Autodesk Fusion 360 part; units mm, degrees
note: some values were not read from the file. Chosen so that the rebuilt part matches the saved one: a direction. Set by a fixed rule: which sketch regions a step uses.
(part 4 of 5)
sketch "Sketch6" plane through (0, 0, 3.1479) normal (0, 0, 1) x (1, 0, 0)
  arc A0 (27.9575, -0.4591) -> (28.2196, 0.5192) centre (23.0613, 1.3771) ccw
  arc A1 (28.3326, 0.6018) -> (28.2196, 0.5192) centre (28.3182, 0.5028) ccw
  line L0 (28.3326, 0.6018) -> (29.1974, 0.4761)
  spline S0 degree 5 poles (29.1974, 0.4761) (29.2018, 0.4754) (29.2105, 0.4743) (29.2236, 0.473) (29.2412, 0.4721) (29.2633, 0.472) (29.2854, 0.4726) (29.3076, 0.4738) (29.3299, 0.4753) (29.3521, 0.4769) (29.3744, 0.4787) (29.3968, 0.4808) (29.4191, 0.4832) (29.4415, 0.486) (29.4639, 0.4891) (29.4863, 0.4927) (29.5087, 0.4965) (29.5311, 0.5006) (29.5536, 0.5049) (29.5761, 0.5095) (29.5985, 0.5143) (29.621, 0.5193) (29.6435, 0.5245) (29.666, 0.53) (29.6885, 0.5357) (29.711, 0.5417) (29.7335, 0.5479) (29.756, 0.5543) (29.7785, 0.561) (29.801, 0.5678) (29.8235, 0.5748) (29.846, 0.5821) (29.8684, 0.5895) (29.8909, 0.5972) (29.9134, 0.605) (29.9359, 0.6131) (29.9583, 0.6213) (29.9808, 0.6298) (30.0032, 0.6384) (30.0256, 0.6472) (30.048, 0.6562) (30.0704, 0.6654) (30.0928, 0.6748) (30.1152, 0.6843) (30.1375, 0.6941) (30.1598, 0.704) (30.1822, 0.7141) (30.2044, 0.7244) (30.2267, 0.7348) (30.249, 0.7455) (30.2712, 0.7563) (30.2934, 0.7672) (30.3156, 0.7784) (30.3378, 0.7897) (30.3599, 0.8012) (30.3821, 0.8128) (30.4042, 0.8246) (30.4262, 0.8366) (30.4483, 0.8488) (30.4703, 0.8611) (30.4923, 0.8736) (30.5142, 0.8862) (30.5362, 0.899) (30.5581, 0.912) (30.5799, 0.9251) (30.6018, 0.9384) (30.6236, 0.9518) (30.6454, 0.9654) (30.6671, 0.9791) (30.6888, 0.9931) (30.7105, 1.0071) (30.7278, 1.0185) (30.7407, 1.0271) (30.7494, 1.0329) (30.7537, 1.0357) knots 0 0 0 0 0 0 0.01428571 0.02857143 0.04285714 0.05714286 0.07142857 0.08571429 0.1 0.11428571 0.12857143 0.14285714 0.15714286 0.17142857 0.18571429 0.2 0.21428571 0.22857143 0.24285714 0.25714286 0.27142857 0.28571429 0.3 0.31428571 0.32857143 0.34285714 0.35714286 0.37142857 0.38571429 0.4 0.41428571 0.42857143 0.44285714 0.45714286 0.47142857 0.48571429 0.5 0.51428571 0.52857143 0.54285714 0.55714286 0.57142857 0.58571429 0.6 0.61428571 0.62857143 0.64285714 0.65714286 0.67142857 0.68571429 0.7 0.71428571 0.72857143 0.74285714 0.75714286 0.77142857 0.78571429 0.8 0.81428571 0.82857143 0.84285714 0.85714286 0.87142857 0.88571429 0.9 0.91428571 0.92857143 0.94285714 0.95714286 0.97142857 0.98571429 1 1 1 1 1 1
  arc A2 (30.7537, 1.0357) -> (30.7537, 1.7185) centre (23.0613, 1.3771) ccw
  spline S1 degree 5 poles (30.7537, 1.7185) (30.7494, 1.7214) (30.7407, 1.7272) (30.7278, 1.7358) (30.7105, 1.7471) (30.6888, 1.7612) (30.6671, 1.7751) (30.6454, 1.7889) (30.6236, 1.8025) (30.6018, 1.8159) (30.5799, 1.8292) (30.5581, 1.8423) (30.5362, 1.8553) (30.5142, 1.8681) (30.4923, 1.8807) (30.4703, 1.8932) (30.4483, 1.9055) (30.4262, 1.9176) (30.4042, 1.9296) (30.3821, 1.9414) (30.3599, 1.9531) (30.3378, 1.9646) (30.3156, 1.9759) (30.2934, 1.987) (30.2712, 1.998) (30.249, 2.0088) (30.2267, 2.0194) (30.2044, 2.0299) (30.1822, 2.0401) (30.1598, 2.0502) (30.1375, 2.0602) (30.1152, 2.0699) (30.0928, 2.0795) (30.0704, 2.0888) (30.048, 2.098) (30.0256, 2.107) (30.0032, 2.1159) (29.9808, 2.1245) (29.9583, 2.1329) (29.9359, 2.1412) (29.9134, 2.1492) (29.8909, 2.1571) (29.8684, 2.1647) (29.846, 2.1722) (29.8235, 2.1794) (29.801, 2.1864) (29.7785, 2.1933) (29.756, 2.1999) (29.7335, 2.2063) (29.711, 2.2125) (29.6885, 2.2185) (29.666, 2.2242) (29.6435, 2.2297) (29.621, 2.235) (29.5985, 2.24) (29.5761, 2.2448) (29.5536, 2.2493) (29.5311, 2.2536) (29.5087, 2.2577) (29.4863, 2.2616) (29.4639, 2.2651) (29.4415, 2.2683) (29.4191, 2.2711) (29.3968, 2.2735) (29.3744, 2.2755) (29.3521, 2.2774) (29.3299, 2.279) (29.3076, 2.2804) (29.2854, 2.2816) (29.2633, 2.2823) (29.2412, 2.2822) (29.2236, 2.2813) (29.2105, 2.28) (29.2018, 2.2788) (29.1974, 2.2782) knots -1 -1 -1 -1 -1 -1 -0.98571429 -0.97142857 -0.95714286 -0.94285714 -0.92857143 -0.91428571 -0.9 -0.88571429 -0.87142857 -0.85714286 -0.84285714 -0.82857143 -0.81428571 -0.8 -0.78571429 -0.77142857 -0.75714286 -0.74285714 -0.72857143 -0.71428571 -0.7 -0.68571429 -0.67142857 -0.65714286 -0.64285714 -0.62857143 -0.61428571 -0.6 -0.58571429 -0.57142857 -0.55714286 -0.54285714 -0.52857143 -0.51428571 -0.5 -0.48571429 -0.47142857 -0.45714286 -0.44285714 -0.42857143 -0.41428571 -0.4 -0.38571429 -0.37142857 -0.35714286 -0.34285714 -0.32857143 -0.31428571 -0.3 -0.28571429 -0.27142857 -0.25714286 -0.24285714 -0.22857143 -0.21428571 -0.2 -0.18571429 -0.17142857 -0.15714286 -0.14285714 -0.12857143 -0.11428571 -0.1 -0.08571429 -0.07142857 -0.05714286 -0.04285714 -0.02857143 -0.01428571 0 0 0 0 0 0
  line L1 (29.1974, 2.2782) -> (28.3326, 2.1525)
  arc A3 (28.2196, 2.2351) -> (28.3326, 2.1525) centre (28.3182, 2.2515) ccw
  arc A4 (28.2196, 2.2351) -> (27.9575, 3.2133) centre (23.0613, 1.3771) ccw
  arc A5 (28.0141, 3.3413) -> (27.9575, 3.2133) centre (28.0511, 3.2484) ccw
  line L2 (28.0141, 3.3413) -> (28.8259, 3.6649)
  spline S2 degree 5 poles (28.8259, 3.6649) (28.83, 3.6665) (28.8381, 3.6699) (28.8501, 3.6753) (28.8658, 3.6833) (28.885, 3.6943) (28.9038, 3.7059) (28.9224, 3.718) (28.941, 3.7304) (28.9594, 3.7429) (28.9778, 3.7557) (28.9961, 3.7686) (29.0143, 3.7819) (29.0323, 3.7955) (29.0501, 3.8094) (29.0677, 3.8237) (29.0852, 3.8382) (29.1026, 3.853) (29.1199, 3.868) (29.1371, 3.8831) (29.1541, 3.8985) (29.1711, 3.9141) (29.1879, 3.9299) (29.2047, 3.9459) (29.2213, 3.9621) (29.2378, 3.9785) (29.2542, 3.9951) (29.2704, 4.0119) (29.2866, 4.0289) (29.3027, 4.0461) (29.3186, 4.0634) (29.3345, 4.081) (29.3502, 4.0986) (29.3659, 4.1165) (29.3814, 4.1345) (29.3969, 4.1527) (29.4122, 4.1711) (29.4274, 4.1896) (29.4425, 4.2083) (29.4575, 4.2272) (29.4724, 4.2462) (29.4872, 4.2653) (29.5019, 4.2847) (29.5165, 4.3041) (29.531, 4.3237) (29.5454, 4.3435) (29.5596, 4.3634) (29.5738, 4.3834) (29.5879, 4.4036) (29.6018, 4.424) (29.6157, 4.4444) (29.6295, 4.465) (29.6431, 4.4858) (29.6566, 4.5067) (29.6701, 4.5277) (29.6834, 4.5488) (29.6966, 4.5701) (29.7098, 4.5915) (29.7228, 4.6131) (29.7357, 4.6347) (29.7485, 4.6565) (29.7612, 4.6785) (29.7738, 4.7005) (29.7863, 4.7227) (29.7986, 4.745) (29.8109, 4.7674) (29.8231, 4.7899) (29.8351, 4.8126) (29.8471, 4.8354) (29.8589, 4.8583) (29.8707, 4.8813) (29.88, 4.8998) (29.8869, 4.9137) (29.8915, 4.923) (29.8938, 4.9277) knots 0 0 0 0 0 0 0.01428571 0.02857143 0.04285714 0.05714286 0.07142857 0.08571429 0.1 0.11428571 0.12857143 0.14285714 0.15714286 0.17142857 0.18571429 0.2 0.21428571 0.22857143 0.24285714 0.25714286 0.27142857 0.28571429 0.3 0.31428571 0.32857143 0.34285714 0.35714286 0.37142857 0.38571429 0.4 0.41428571 0.42857143 0.44285714 0.45714286 0.47142857 0.48571429 0.5 0.51428571 0.52857143 0.54285714 0.55714286 0.57142857 0.58571429 0.6 0.61428571 0.62857143 0.64285714 0.65714286 0.67142857 0.68571429 0.7 0.71428571 0.72857143 0.74285714 0.75714286 0.77142857 0.78571429 0.8 0.81428571 0.82857143 0.84285714 0.85714286 0.87142857 0.88571429 0.9 0.91428571 0.92857143 0.94285714 0.95714286 0.97142857 0.98571429 1 1 1 1 1 1
  arc A6 (29.8938, 4.9277) -> (29.5524, 5.519) centre (23.0613, 1.3771) ccw
  spline S3 degree 5 poles (29.5524, 5.519) (29.5472, 5.5193) (29.5369, 5.52) (29.5213, 5.521) (29.5007, 5.5222) (29.4749, 5.5235) (29.4491, 5.5247) (29.4234, 5.5257) (29.3978, 5.5266) (29.3722, 5.5274) (29.3466, 5.528) (29.3211, 5.5284) (29.2957, 5.5287) (29.2703, 5.5288) (29.2449, 5.5287) (29.2197, 5.5286) (29.1944, 5.5282) (29.1693, 5.5277) (29.1442, 5.5271) (29.1191, 5.5262) (29.0941, 5.5253) (29.0692, 5.5241) (29.0444, 5.5228) (29.0196, 5.5214) (28.9948, 5.5198) (28.9702, 5.518) (28.9456, 5.5161) (28.9211, 5.514) (28.8966, 5.5118) (28.8722, 5.5094) (28.8479, 5.5068) (28.8237, 5.504) (28.7996, 5.5011) (28.7755, 5.4981) (28.7515, 5.4948) (28.7276, 5.4914) (28.7038, 5.4878) (28.68, 5.4841) (28.6564, 5.4802) (28.6328, 5.4761) (28.6093, 5.4718) (28.5859, 5.4674) (28.5627, 5.4628) (28.5395, 5.458) (28.5164, 5.453) (28.4934, 5.4479) (28.4705, 5.4426) (28.4477, 5.437) (28.425, 5.4314) (28.4024, 5.4255) (28.3799, 5.4194) (28.3576, 5.4131) (28.3353, 5.4066) (28.3132, 5.3999) (28.2913, 5.393) (28.2694, 5.3859) (28.2477, 5.3786) (28.2261, 5.3712) (28.2046, 5.3635) (28.1832, 5.3556) (28.1621, 5.3474) (28.1411, 5.339) (28.1203, 5.3302) (28.0998, 5.3211) (28.0794, 5.3118) (28.0592, 5.3022) (28.0391, 5.2925) (28.0191, 5.2826) (27.9993, 5.2725) (27.9798, 5.262) (27.9607, 5.2509) (27.946, 5.2413) (27.9352, 5.2336) (27.9282, 5.2283) (27.9248, 5.2256) knots -1 -1 -1 -1 -1 -1 -0.98571429 -0.97142857 -0.95714286 -0.94285714 -0.92857143 -0.91428571 -0.9 -0.88571429 -0.87142857 -0.85714286 -0.84285714 -0.82857143 -0.81428571 -0.8 -0.78571429 -0.77142857 -0.75714286 -0.74285714 -0.72857143 -0.71428571 -0.7 -0.68571429 -0.67142857 -0.65714286 -0.64285714 -0.62857143 -0.61428571 -0.6 -0.58571429 -0.57142857 -0.55714286 -0.54285714 -0.52857143 -0.51428571 -0.5 -0.48571429 -0.47142857 -0.45714286 -0.44285714 -0.42857143 -0.41428571 -0.4 -0.38571429 -0.37142857 -0.35714286 -0.34285714 -0.32857143 -0.31428571 -0.3 -0.28571429 -0.27142857 -0.25714286 -0.24285714 -0.22857143 -0.21428571 -0.2 -0.18571429 -0.17142857 -0.15714286 -0.14285714 -0.12857143 -0.11428571 -0.1 -0.08571429 -0.07142857 -0.05714286 -0.04285714 -0.02857143 -0.01428571 0 0 0 0 0 0
  line L3 (27.9248, 5.2256) -> (27.2387, 4.6843)
  arc A7 (27.0995, 4.6993) -> (27.2387, 4.6843) centre (27.1768, 4.7628) ccw
  arc A8 (27.0995, 4.6993) -> (26.3834, 5.4154) centre (23.0613, 1.3771) ccw
  arc A9 (26.3684, 5.5546) -> (26.3834, 5.4154) centre (26.4469, 5.4926) ccw
  line L4 (26.3684, 5.5546) -> (26.9097, 6.2407)
  spline S4 degree 5 poles (26.9097, 6.2407) (26.9124, 6.2441) (26.9178, 6.2511) (26.9254, 6.2619) (26.935, 6.2766) (26.9462, 6.2957) (26.9566, 6.3152) (26.9667, 6.335) (26.9766, 6.355) (26.9863, 6.3751) (26.9959, 6.3953) (27.0053, 6.4157) (27.0144, 6.4362) (27.0231, 6.457) (27.0316, 6.4779) (27.0397, 6.4991) (27.0476, 6.5205) (27.0553, 6.542) (27.0628, 6.5636) (27.07, 6.5853) (27.0771, 6.6071) (27.0841, 6.6291) (27.0908, 6.6512) (27.0972, 6.6734) (27.1035, 6.6958) (27.1096, 6.7183) (27.1155, 6.7408) (27.1212, 6.7635) (27.1267, 6.7863) (27.132, 6.8092) (27.1372, 6.8322) (27.1421, 6.8553) (27.1469, 6.8785) (27.1515, 6.9018) (27.156, 6.9252) (27.1602, 6.9487) (27.1643, 6.9723) (27.1682, 6.9959) (27.172, 7.0197) (27.1755, 7.0435) (27.179, 7.0674) (27.1822, 7.0914) (27.1853, 7.1154) (27.1882, 7.1396) (27.1909, 7.1638) (27.1935, 7.1881) (27.1959, 7.2125) (27.1981, 7.2369) (27.2002, 7.2615) (27.2022, 7.2861) (27.2039, 7.3107) (27.2055, 7.3354) (27.207, 7.3602) (27.2083, 7.3851) (27.2094, 7.41) (27.2104, 7.435) (27.2112, 7.46) (27.2118, 7.4851) (27.2123, 7.5103) (27.2127, 7.5355) (27.2129, 7.5608) (27.2129, 7.5861) (27.2128, 7.6115) (27.2125, 7.637) (27.2121, 7.6625) (27.2115, 7.688) (27.2108, 7.7136) (27.2099, 7.7393) (27.2088, 7.765) (27.2076, 7.7907) (27.2063, 7.8165) (27.2051, 7.8372) (27.2041, 7.8527) (27.2035, 7.8631) (27.2031, 7.8683) knots 0 0 0 0 0 0 0.01428571 0.02857143 0.04285714 0.05714286 0.07142857 0.08571429 0.1 0.11428571 0.12857143 0.14285714 0.15714286 0.17142857 0.18571429 0.2 0.21428571 0.22857143 0.24285714 0.25714286 0.27142857 0.28571429 0.3 0.31428571 0.32857143 0.34285714 0.35714286 0.37142857 0.38571429 0.4 0.41428571 0.42857143 0.44285714 0.45714286 0.47142857 0.48571429 0.5 0.51428571 0.52857143 0.54285714 0.55714286 0.57142857 0.58571429 0.6 0.61428571 0.62857143 0.64285714 0.65714286 0.67142857 0.68571429 0.7 0.71428571 0.72857143 0.74285714 0.75714286 0.77142857 0.78571429 0.8 0.81428571 0.82857143 0.84285714 0.85714286 0.87142857 0.88571429 0.9 0.91428571 0.92857143 0.94285714 0.95714286 0.97142857 0.98571429 1 1 1 1 1 1
  arc A10 (27.2031, 7.8683) -> (26.6118, 8.2097) centre (23.0613, 1.3771) ccw
  spline S5 degree 5 poles (26.6118, 8.2097) (26.6072, 8.2074) (26.5978, 8.2028) (26.5839, 8.1958) (26.5654, 8.1865) (26.5424, 8.1748) (26.5195, 8.163) (26.4967, 8.151) (26.4741, 8.139) (26.4515, 8.1268) (26.4291, 8.1145) (26.4068, 8.1021) (26.3846, 8.0897) (26.3626, 8.0771) (26.3407, 8.0644) (26.3189, 8.0516) (26.2972, 8.0387) (26.2757, 8.0256) (26.2542, 8.0125) (26.233, 7.9993) (26.2118, 7.986) (26.1908, 7.9725) (26.1699, 7.959) (26.1492, 7.9453) (26.1286, 7.9316) (26.1081, 7.9177) (26.0877, 7.9038) (26.0676, 7.8897) (26.0475, 7.8755) (26.0276, 7.8612) (26.0078, 7.8469) (25.9882, 7.8324) (25.9688, 7.8178) (25.9495, 7.8031) (25.9303, 7.7883) (25.9113, 7.7734) (25.8925, 7.7584) (25.8738, 7.7433) (25.8552, 7.728) (25.8369, 7.7127) (25.8187, 7.6973) (25.8006, 7.6818) (25.7828, 7.6661) (25.7651, 7.6504) (25.7476, 7.6345) (25.7302, 7.6186) (25.7131, 7.6025) (25.6961, 7.5863) (25.6793, 7.57) (25.6626, 7.5537) (25.6462, 7.5372) (25.63, 7.5206) (25.614, 7.5038) (25.5982, 7.487) (25.5826, 7.47) (25.5673, 7.4529) (25.5521, 7.4357) (25.5371, 7.4185) (25.5223, 7.4011) (25.5078, 7.3836) (25.4935, 7.3659) (25.4796, 7.3481) (25.466, 7.3302) (25.4527, 7.312) (25.4398, 7.2937) (25.4271, 7.2753) (25.4145, 7.2569) (25.4022, 7.2383) (25.39, 7.2197) (25.3784, 7.2008) (25.3674, 7.1817) (25.3595, 7.166) (25.354, 7.154) (25.3506, 7.1458) (25.349, 7.1417) knots -1 -1 -1 -1 -1 -1 -0.98571429 -0.97142857 -0.95714286 -0.94285714 -0.92857143 -0.91428571 -0.9 -0.88571429 -0.87142857 -0.85714286 -0.84285714 -0.82857143 -0.81428571 -0.8 -0.78571429 -0.77142857 -0.75714286 -0.74285714 -0.72857143 -0.71428571 -0.7 -0.68571429 -0.67142857 -0.65714286 -0.64285714 -0.62857143 -0.61428571 -0.6 -0.58571429 -0.57142857 -0.55714286 -0.54285714 -0.52857143 -0.51428571 -0.5 -0.48571429 -0.47142857 -0.45714286 -0.44285714 -0.42857143 -0.41428571 -0.4 -0.38571429 -0.37142857 -0.35714286 -0.34285714 -0.32857143 -0.31428571 -0.3 -0.28571429 -0.27142857 -0.25714286 -0.24285714 -0.22857143 -0.21428571 -0.2 -0.18571429 -0.17142857 -0.15714286 -0.14285714 -0.12857143 -0.11428571 -0.1 -0.08571429 -0.07142857 -0.05714286 -0.04285714 -0.02857143 -0.01428571 0 0 0 0 0 0
  line L5 (25.349, 7.1417) -> (25.0254, 6.33)
  arc A11 (24.8974, 6.2733) -> (25.0254, 6.33) centre (24.9326, 6.367) ccw
  arc A12 (24.8974, 6.2733) -> (23.9192, 6.5355) centre (23.0613, 1.3771) ccw
  arc A13 (23.8366, 6.6485) -> (23.9192, 6.5355) centre (23.9356, 6.6341) ccw
  line L6 (23.8366, 6.6485) -> (23.9623, 7.5133)
  spline S6 degree 5 poles (23.9623, 7.5133) (23.963, 7.5177) (23.9641, 7.5264) (23.9654, 7.5395) (23.9663, 7.5571) (23.9664, 7.5792) (23.9657, 7.6013) (23.9646, 7.6235) (23.9631, 7.6458) (23.9615, 7.668) (23.9597, 7.6903) (23.9576, 7.7126) (23.9552, 7.735) (23.9524, 7.7573) (23.9492, 7.7797) (23.9457, 7.8021) (23.9419, 7.8246) (23.9378, 7.847) (23.9334, 7.8695) (23.9289, 7.8919) (23.9241, 7.9144) (23.9191, 7.9369) (23.9139, 7.9594) (23.9084, 7.9819) (23.9026, 8.0044) (23.8967, 8.0269) (23.8905, 8.0494) (23.884, 8.0719) (23.8774, 8.0944) (23.8706, 8.1169) (23.8635, 8.1393) (23.8563, 8.1618) (23.8488, 8.1843) (23.8412, 8.2068) (23.8333, 8.2293) (23.8253, 8.2517) (23.817, 8.2742) (23.8086, 8.2966) (23.8, 8.3191) (23.7912, 8.3415) (23.7822, 8.3639) (23.773, 8.3863) (23.7636, 8.4087) (23.754, 8.431) (23.7443, 8.4534) (23.7344, 8.4757) (23.7243, 8.498) (23.714, 8.5203) (23.7035, 8.5426) (23.6929, 8.5649) (23.6821, 8.5871) (23.6711, 8.6093) (23.66, 8.6315) (23.6487, 8.6537) (23.6372, 8.6758) (23.6256, 8.6979) (23.6137, 8.72) (23.6018, 8.7421) (23.5896, 8.7642) (23.5773, 8.7862) (23.5648, 8.8082) (23.5522, 8.8301) (23.5394, 8.852) (23.5264, 8.8739) (23.5133, 8.8958) (23.5, 8.9177) (23.4866, 8.9395) (23.473, 8.9612) (23.4592, 8.983) (23.4453, 9.0047) (23.4313, 9.0263) (23.4199, 9.0436) (23.4113, 9.0566) (23.4055, 9.0652) (23.4026, 9.0696) knots 0 0 0 0 0 0 0.01428571 0.02857143 0.04285714 0.05714286 0.07142857 0.08571429 0.1 0.11428571 0.12857143 0.14285714 0.15714286 0.17142857 0.18571429 0.2 0.21428571 0.22857143 0.24285714 0.25714286 0.27142857 0.28571429 0.3 0.31428571 0.32857143 0.34285714 0.35714286 0.37142857 0.38571429 0.4 0.41428571 0.42857143 0.44285714 0.45714286 0.47142857 0.48571429 0.5 0.51428571 0.52857143 0.54285714 0.55714286 0.57142857 0.58571429 0.6 0.61428571 0.62857143 0.64285714 0.65714286 0.67142857 0.68571429 0.7 0.71428571 0.72857143 0.74285714 0.75714286 0.77142857 0.78571429 0.8 0.81428571 0.82857143 0.84285714 0.85714286 0.87142857 0.88571429 0.9 0.91428571 0.92857143 0.94285714 0.95714286 0.97142857 0.98571429 1 1 1 1 1 1
  arc A14 (23.4026, 9.0696) -> (22.7199, 9.0696) centre (23.0613, 1.3771) ccw
  spline S7 degree 5 poles (22.7199, 9.0696) (22.717, 9.0652) (22.7112, 9.0566) (22.7026, 9.0436) (22.6912, 9.0263) (22.6772, 9.0047) (22.6633, 8.983) (22.6495, 8.9612) (22.6359, 8.9395) (22.6225, 8.9177) (22.6092, 8.8958) (22.5961, 8.8739) (22.5831, 8.852) (22.5703, 8.8301) (22.5577, 8.8082) (22.5452, 8.7862) (22.5329, 8.7642) (22.5207, 8.7421) (22.5088, 8.72) (22.4969, 8.6979) (22.4853, 8.6758) (22.4738, 8.6537) (22.4625, 8.6315) (22.4514, 8.6093) (22.4404, 8.5871) (22.4296, 8.5649) (22.419, 8.5426) (22.4085, 8.5203) (22.3982, 8.498) (22.3881, 8.4757) (22.3782, 8.4534) (22.3685, 8.431) (22.3589, 8.4087) (22.3495, 8.3863) (22.3403, 8.3639) (22.3313, 8.3415) (22.3225, 8.3191) (22.3139, 8.2966) (22.3055, 8.2742) (22.2972, 8.2517) (22.2892, 8.2293) (22.2813, 8.2068) (22.2737, 8.1843) (22.2662, 8.1618) (22.259, 8.1393) (22.2519, 8.1169) (22.2451, 8.0944) (22.2385, 8.0719) (22.232, 8.0494) (22.2258, 8.0269) (22.2199, 8.0044) (22.2141, 7.9819) (22.2086, 7.9594) (22.2034, 7.9369) (22.1984, 7.9144) (22.1936, 7.8919) (22.1891, 7.8695) (22.1847, 7.847) (22.1806, 7.8246) (22.1768, 7.8021) (22.1733, 7.7797) (22.1701, 7.7573) (22.1673, 7.735) (22.1649, 7.7126) (22.1628, 7.6903) (22.161, 7.668) (22.1594, 7.6458) (22.1579, 7.6235) (22.1568, 7.6013) (22.1561, 7.5792) (22.1562, 7.5571) (22.1571, 7.5395) (22.1584, 7.5264) (22.1595, 7.5177) (22.1602, 7.5133) knots -1 -1 -1 -1 -1 -1 -0.98571429 -0.97142857 -0.95714286 -0.94285714 -0.92857143 -0.91428571 -0.9 -0.88571429 -0.87142857 -0.85714286 -0.84285714 -0.82857143 -0.81428571 -0.8 -0.78571429 -0.77142857 -0.75714286 -0.74285714 -0.72857143 -0.71428571 -0.7 -0.68571429 -0.67142857 -0.65714286 -0.64285714 -0.62857143 -0.61428571 -0.6 -0.58571429 -0.57142857 -0.55714286 -0.54285714 -0.52857143 -0.51428571 -0.5 -0.48571429 -0.47142857 -0.45714286 -0.44285714 -0.42857143 -0.41428571 -0.4 -0.38571429 -0.37142857 -0.35714286 -0.34285714 -0.32857143 -0.31428571 -0.3 -0.28571429 -0.27142857 -0.25714286 -0.24285714 -0.22857143 -0.21428571 -0.2 -0.18571429 -0.17142857 -0.15714286 -0.14285714 -0.12857143 -0.11428571 -0.1 -0.08571429 -0.07142857 -0.05714286 -0.04285714 -0.02857143 -0.01428571 0 0 0 0 0 0
  line L7 (22.1602, 7.5133) -> (22.2859, 6.6485)
  arc A15 (22.2033, 6.5355) -> (22.2859, 6.6485) centre (22.1869, 6.6341) ccw
  arc A16 (22.2033, 6.5355) -> (21.2251, 6.2733) centre (23.0613, 1.3771) ccw
  arc A17 (21.0971, 6.33) -> (21.2251, 6.2733) centre (21.19, 6.367) ccw
  line L8 (21.0971, 6.33) -> (20.7735, 7.1417)
  spline S8 degree 5 poles (20.7735, 7.1417) (20.7719, 7.1458) (20.7685, 7.154) (20.763, 7.166) (20.7551, 7.1817) (20.7441, 7.2008) (20.7325, 7.2197) (20.7203, 7.2383) (20.708, 7.2569) (20.6954, 7.2753) (20.6827, 7.2937) (20.6698, 7.312) (20.6565, 7.3302) (20.6429, 7.3481) (20.629, 7.3659) (20.6147, 7.3836) (20.6002, 7.4011) (20.5854, 7.4185) (20.5704, 7.4357) (20.5552, 7.4529) (20.5399, 7.47) (20.5243, 7.487) (20.5085, 7.5038) (20.4925, 7.5206) (20.4763, 7.5372) (20.4599, 7.5537) (20.4432, 7.57) (20.4264, 7.5863) (20.4094, 7.6025) (20.3923, 7.6186) (20.3749, 7.6345) (20.3574, 7.6504) (20.3397, 7.6661) (20.3219, 7.6818) (20.3038, 7.6973) (20.2856, 7.7127) (20.2673, 7.728) (20.2487, 7.7433) (20.23, 7.7584) (20.2112, 7.7734) (20.1922, 7.7883) (20.173, 7.8031) (20.1537, 7.8178) (20.1343, 7.8324) (20.1147, 7.8469) (20.0949, 7.8612) (20.075, 7.8755) (20.0549, 7.8897) (20.0348, 7.9038) (20.0144, 7.9177) (19.994, 7.9316) (19.9733, 7.9453) (19.9526, 7.959) (19.9317, 7.9725) (19.9107, 7.986) (19.8895, 7.9993) (19.8683, 8.0125) (19.8468, 8.0256) (19.8253, 8.0387) (19.8036, 8.0516) (19.7818, 8.0644) (19.7599, 8.0771) (19.7379, 8.0897) (19.7157, 8.1021) (19.6934, 8.1145) (19.671, 8.1268) (19.6484, 8.139) (19.6258, 8.151) (19.603, 8.163) (19.5801, 8.1748) (19.5571, 8.1865) (19.5386, 8.1958) (19.5247, 8.2028) (19.5153, 8.2074) (19.5107, 8.2097) knots 0 0 0 0 0 0 0.01428571 0.02857143 0.04285714 0.05714286 0.07142857 0.08571429 0.1 0.11428571 0.12857143 0.14285714 0.15714286 0.17142857 0.18571429 0.2 0.21428571 0.22857143 0.24285714 0.25714286 0.27142857 0.28571429 0.3 0.31428571 0.32857143 0.34285714 0.35714286 0.37142857 0.38571429 0.4 0.41428571 0.42857143 0.44285714 0.45714286 0.47142857 0.48571429 0.5 0.51428571 0.52857143 0.54285714 0.55714286 0.57142857 0.58571429 0.6 0.61428571 0.62857143 0.64285714 0.65714286 0.67142857 0.68571429 0.7 0.71428571 0.72857143 0.74285714 0.75714286 0.77142857 0.78571429 0.8 0.81428571 0.82857143 0.84285714 0.85714286 0.87142857 0.88571429 0.9 0.91428571 0.92857143 0.94285714 0.95714286 0.97142857 0.98571429 1 1 1 1 1 1
  arc A18 (19.5107, 8.2097) -> (18.9194, 7.8683) centre (23.0613, 1.3771) ccw
  spline S9 degree 5 poles (18.9194, 7.8683) (18.919, 7.8631) (18.9184, 7.8527) (18.9174, 7.8372) (18.9162, 7.8165) (18.9149, 7.7907) (18.9137, 7.765) (18.9126, 7.7393) (18.9117, 7.7136) (18.911, 7.688) (18.9104, 7.6625) (18.91, 7.637) (18.9097, 7.6115) (18.9096, 7.5861) (18.9096, 7.5608) (18.9098, 7.5355) (18.9102, 7.5103) (18.9107, 7.4851) (18.9113, 7.46) (18.9121, 7.435) (18.9131, 7.41) (18.9142, 7.3851) (18.9155, 7.3602) (18.917, 7.3354) (18.9186, 7.3107) (18.9203, 7.2861) (18.9223, 7.2615) (18.9244, 7.2369) (18.9266, 7.2125) (18.929, 7.1881) (18.9316, 7.1638) (18.9343, 7.1396) (18.9372, 7.1154) (18.9403, 7.0914) (18.9436, 7.0674) (18.947, 7.0435) (18.9505, 7.0197) (18.9543, 6.9959) (18.9582, 6.9723) (18.9623, 6.9487) (18.9665, 6.9252) (18.971, 6.9018) (18.9756, 6.8785) (18.9804, 6.8553) (18.9853, 6.8322) (18.9905, 6.8092) (18.9958, 6.7863) (19.0013, 6.7635) (19.007, 6.7408) (19.0129, 6.7183) (19.019, 6.6958) (19.0253, 6.6734) (19.0317, 6.6512) (19.0385, 6.6291) (19.0454, 6.6071) (19.0525, 6.5853) (19.0597, 6.5636) (19.0672, 6.542) (19.0749, 6.5205) (19.0828, 6.4991) (19.0909, 6.4779) (19.0994, 6.457) (19.1081, 6.4362) (19.1172, 6.4157) (19.1266, 6.3953) (19.1362, 6.3751) (19.1459, 6.355) (19.1558, 6.335) (19.1659, 6.3152) (19.1763, 6.2957) (19.1875, 6.2766) (19.1971, 6.2619) (19.2047, 6.2511) (19.2101, 6.2441) (19.2128, 6.2407) knots -1 -1 -1 -1 -1 -1 -0.98571429 -0.97142857 -0.95714286 -0.94285714 -0.92857143 -0.91428571 -0.9 -0.88571429 -0.87142857 -0.85714286 -0.84285714 -0.82857143 -0.81428571 -0.8 -0.78571429 -0.77142857 -0.75714286 -0.74285714 -0.72857143 -0.71428571 -0.7 -0.68571429 -0.67142857 -0.65714286 -0.64285714 -0.62857143 -0.61428571 -0.6 -0.58571429 -0.57142857 -0.55714286 -0.54285714 -0.52857143 -0.51428571 -0.5 -0.48571429 -0.47142857 -0.45714286 -0.44285714 -0.42857143 -0.41428571 -0.4 -0.38571429 -0.37142857 -0.35714286 -0.34285714 -0.32857143 -0.31428571 -0.3 -0.28571429 -0.27142857 -0.25714286 -0.24285714 -0.22857143 -0.21428571 -0.2 -0.18571429 -0.17142857 -0.15714286 -0.14285714 -0.12857143 -0.11428571 -0.1 -0.08571429 -0.07142857 -0.05714286 -0.04285714 -0.02857143 -0.01428571 0 0 0 0 0 0
  line L9 (19.2128, 6.2407) -> (19.7541, 5.5546)
  arc A19 (19.7391, 5.4154) -> (19.7541, 5.5546) centre (19.6756, 5.4926) ccw
  arc A20 (19.7391, 5.4154) -> (19.023, 4.6993) centre (23.0613, 1.3771) ccw
  arc A21 (18.8838, 4.6843) -> (19.023, 4.6993) centre (18.9457, 4.7628) ccw
  line L10 (18.8838, 4.6843) -> (18.1977, 5.2256)
  spline S10 degree 5 poles (18.1977, 5.2256) (18.1943, 5.2283) (18.1873, 5.2336) (18.1765, 5.2413) (18.1618, 5.2509) (18.1427, 5.262) (18.1232, 5.2725) (18.1034, 5.2826) (18.0834, 5.2925) (18.0633, 5.3022) (18.0431, 5.3118) (18.0227, 5.3211) (18.0022, 5.3302) (17.9814, 5.339) (17.9604, 5.3474) (17.9393, 5.3556) (17.9179, 5.3635) (17.8964, 5.3712) (17.8748, 5.3786) (17.8531, 5.3859) (17.8312, 5.393) (17.8093, 5.3999) (17.7872, 5.4066) (17.7649, 5.4131) (17.7426, 5.4194) (17.7201, 5.4255) (17.6975, 5.4314) (17.6748, 5.437) (17.652, 5.4426) (17.6291, 5.4479) (17.6061, 5.453) (17.583, 5.458) (17.5599, 5.4628) (17.5366, 5.4674) (17.5132, 5.4718) (17.4897, 5.4761) (17.4661, 5.4802) (17.4425, 5.4841) (17.4187, 5.4878) (17.3949, 5.4914) (17.371, 5.4948) (17.347, 5.4981) (17.3229, 5.5011) (17.2988, 5.504) (17.2746, 5.5068) (17.2503, 5.5094) (17.2259, 5.5118) (17.2014, 5.514) (17.1769, 5.5161) (17.1523, 5.518) (17.1277, 5.5198) (17.1029, 5.5214) (17.0782, 5.5228) (17.0533, 5.5241) (17.0284, 5.5253) (17.0034, 5.5262) (16.9783, 5.5271) (16.9532, 5.5277) (16.9281, 5.5282) (16.9029, 5.5286) (16.8776, 5.5287) (16.8522, 5.5288) (16.8268, 5.5287) (16.8014, 5.5284) (16.7759, 5.528) (16.7503, 5.5274) (16.7247, 5.5266) (16.6991, 5.5257) (16.6734, 5.5247) (16.6476, 5.5235) (16.6219, 5.5222) (16.6012, 5.521) (16.5856, 5.52) (16.5753, 5.5193) (16.5701, 5.519) knots 0 0 0 0 0 0 0.01428571 0.02857143 0.04285714 0.05714286 0.07142857 0.08571429 0.1 0.11428571 0.12857143 0.14285714 0.15714286 0.17142857 0.18571429 0.2 0.21428571 0.22857143 0.24285714 0.25714286 0.27142857 0.28571429 0.3 0.31428571 0.32857143 0.34285714 0.35714286 0.37142857 0.38571429 0.4 0.41428571 0.42857143 0.44285714 0.45714286 0.47142857 0.48571429 0.5 0.51428571 0.52857143 0.54285714 0.55714286 0.57142857 0.58571429 0.6 0.61428571 0.62857143 0.64285714 0.65714286 0.67142857 0.68571429 0.7 0.71428571 0.72857143 0.74285714 0.75714286 0.77142857 0.78571429 0.8 0.81428571 0.82857143 0.84285714 0.85714286 0.87142857 0.88571429 0.9 0.91428571 0.92857143 0.94285714 0.95714286 0.97142857 0.98571429 1 1 1 1 1 1
  arc A22 (16.5701, 5.519) -> (16.2287, 4.9277) centre (23.0613, 1.3771) ccw
  spline S11 degree 5 poles (16.2287, 4.9277) (16.231, 4.923) (16.2356, 4.9137) (16.2425, 4.8998) (16.2518, 4.8813) (16.2636, 4.8583) (16.2754, 4.8354) (16.2874, 4.8126) (16.2994, 4.7899) (16.3116, 4.7674) (16.3239, 4.745) (16.3362, 4.7227) (16.3487, 4.7005) (16.3613, 4.6785) (16.374, 4.6565) (16.3868, 4.6347) (16.3997, 4.6131) (16.4127, 4.5915) (16.4259, 4.5701) (16.4391, 4.5488) (16.4524, 4.5277) (16.4659, 4.5067) (16.4794, 4.4858) (16.493, 4.465) (16.5068, 4.4444) (16.5207, 4.424) (16.5346, 4.4036) (16.5487, 4.3834) (16.5629, 4.3634) (16.5771, 4.3435) (16.5915, 4.3237) (16.606, 4.3041) (16.6206, 4.2847) (16.6353, 4.2653) (16.6501, 4.2462) (16.665, 4.2272) (16.68, 4.2083) (16.6951, 4.1896) (16.7103, 4.1711) (16.7257, 4.1527) (16.7411, 4.1345) (16.7566, 4.1165) (16.7723, 4.0986) (16.788, 4.081) (16.8039, 4.0634) (16.8198, 4.0461) (16.8359, 4.0289) (16.8521, 4.0119) (16.8683, 3.9951) (16.8847, 3.9785) (16.9012, 3.9621) (16.9178, 3.9459) (16.9346, 3.9299) (16.9514, 3.9141) (16.9684, 3.8985) (16.9855, 3.8831) (17.0026, 3.868) (17.0199, 3.853) (17.0373, 3.8382) (17.0548, 3.8237) (17.0724, 3.8094) (17.0902, 3.7955) (17.1082, 3.7819) (17.1264, 3.7686) (17.1447, 3.7557) (17.1631, 3.7429) (17.1815, 3.7304) (17.2001, 3.718) (17.2187, 3.7059) (17.2375, 3.6943) (17.2567, 3.6833) (17.2724, 3.6753) (17.2844, 3.6699) (17.2925, 3.6665) (17.2966, 3.6649) knots -1 -1 -1 -1 -1 -1 -0.98571429 -0.97142857 -0.95714286 -0.94285714 -0.92857143 -0.91428571 -0.9 -0.88571429 -0.87142857 -0.85714286 -0.84285714 -0.82857143 -0.81428571 -0.8 -0.78571429 -0.77142857 -0.75714286 -0.74285714 -0.72857143 -0.71428571 -0.7 -0.68571429 -0.67142857 -0.65714286 -0.64285714 -0.62857143 -0.61428571 -0.6 -0.58571429 -0.57142857 -0.55714286 -0.54285714 -0.52857143 -0.51428571 -0.5 -0.48571429 -0.47142857 -0.45714286 -0.44285714 -0.42857143 -0.41428571 -0.4 -0.38571429 -0.37142857 -0.35714286 -0.34285714 -0.32857143 -0.31428571 -0.3 -0.28571429 -0.27142857 -0.25714286 -0.24285714 -0.22857143 -0.21428571 -0.2 -0.18571429 -0.17142857 -0.15714286 -0.14285714 -0.12857143 -0.11428571 -0.1 -0.08571429 -0.07142857 -0.05714286 -0.04285714 -0.02857143 -0.01428571 0 0 0 0 0 0
  line L11 (17.2966, 3.6649) -> (18.1084, 3.3413)
  arc A23 (18.165, 3.2133) -> (18.1084, 3.3413) centre (18.0714, 3.2484) ccw
  arc A24 (18.165, 3.2133) -> (17.9029, 2.2351) centre (23.0613, 1.3771) ccw
  arc A25 (17.7899, 2.1525) -> (17.9029, 2.2351) centre (17.8043, 2.2515) ccw
  line L12 (17.7899, 2.1525) -> (16.9251, 2.2782)
  spline S12 degree 5 poles (16.9251, 2.2782) (16.9207, 2.2788) (16.912, 2.28) (16.8989, 2.2813) (16.8813, 2.2822) (16.8592, 2.2823) (16.8371, 2.2816) (16.8149, 2.2804) (16.7926, 2.279) (16.7704, 2.2774) (16.7481, 2.2755) (16.7258, 2.2735) (16.7034, 2.2711) (16.681, 2.2683) (16.6587, 2.2651) (16.6362, 2.2616) (16.6138, 2.2577) (16.5914, 2.2536) (16.5689, 2.2493) (16.5464, 2.2448) (16.524, 2.24) (16.5015, 2.235) (16.479, 2.2297) (16.4565, 2.2242) (16.434, 2.2185) (16.4115, 2.2125) (16.389, 2.2063) (16.3665, 2.1999) (16.344, 2.1933) (16.3215, 2.1864) (16.299, 2.1794) (16.2765, 2.1722) (16.2541, 2.1647) (16.2316, 2.1571) (16.2091, 2.1492) (16.1867, 2.1412) (16.1642, 2.1329) (16.1418, 2.1245) (16.1193, 2.1159) (16.0969, 2.107) (16.0745, 2.098) (16.0521, 2.0888) (16.0297, 2.0795) (16.0073, 2.0699) (15.985, 2.0602) (15.9627, 2.0502) (15.9404, 2.0401) (15.9181, 2.0299) (15.8958, 2.0194) (15.8735, 2.0088) (15.8513, 1.998) (15.8291, 1.987) (15.8069, 1.9759) (15.7847, 1.9646) (15.7626, 1.9531) (15.7404, 1.9414) (15.7183, 1.9296) (15.6963, 1.9176) (15.6742, 1.9055) (15.6522, 1.8932) (15.6302, 1.8807) (15.6083, 1.8681) (15.5863, 1.8553) (15.5644, 1.8423) (15.5426, 1.8292) (15.5207, 1.8159) (15.4989, 1.8025) (15.4772, 1.7889) (15.4554, 1.7751) (15.4337, 1.7612) (15.412, 1.7471) (15.3947, 1.7358) (15.3818, 1.7272) (15.3731, 1.7214) (15.3688, 1.7185) knots 0 0 0 0 0 0 0.01428571 0.02857143 0.04285714 0.05714286 0.07142857 0.08571429 0.1 0.11428571 0.12857143 0.14285714 0.15714286 0.17142857 0.18571429 0.2 0.21428571 0.22857143 0.24285714 0.25714286 0.27142857 0.28571429 0.3 0.31428571 0.32857143 0.34285714 0.35714286 0.37142857 0.38571429 0.4 0.41428571 0.42857143 0.44285714 0.45714286 0.47142857 0.48571429 0.5 0.51428571 0.52857143 0.54285714 0.55714286 0.57142857 0.58571429 0.6 0.61428571 0.62857143 0.64285714 0.65714286 0.67142857 0.68571429 0.7 0.71428571 0.72857143 0.74285714 0.75714286 0.77142857 0.78571429 0.8 0.81428571 0.82857143 0.84285714 0.85714286 0.87142857 0.88571429 0.9 0.91428571 0.92857143 0.94285714 0.95714286 0.97142857 0.98571429 1 1 1 1 1 1
  arc A26 (15.3688, 1.7185) -> (15.3688, 1.0357) centre (23.0613, 1.3771) ccw
  spline S13 degree 5 poles (15.3688, 1.0357) (15.3731, 1.0329) (15.3818, 1.0271) (15.3947, 1.0185) (15.412, 1.0071) (15.4337, 0.9931) (15.4554, 0.9791) (15.4772, 0.9654) (15.4989, 0.9518) (15.5207, 0.9384) (15.5426, 0.9251) (15.5644, 0.912) (15.5863, 0.899) (15.6083, 0.8862) (15.6302, 0.8736) (15.6522, 0.8611) (15.6742, 0.8488) (15.6963, 0.8366) (15.7183, 0.8246) (15.7404, 0.8128) (15.7626, 0.8012) (15.7847, 0.7897) (15.8069, 0.7784) (15.8291, 0.7672) (15.8513, 0.7563) (15.8735, 0.7455) (15.8958, 0.7348) (15.9181, 0.7244) (15.9404, 0.7141) (15.9627, 0.704) (15.985, 0.6941) (16.0073, 0.6843) (16.0297, 0.6748) (16.0521, 0.6654) (16.0745, 0.6562) (16.0969, 0.6472) (16.1193, 0.6384) (16.1418, 0.6298) (16.1642, 0.6213) (16.1867, 0.6131) (16.2091, 0.605) (16.2316, 0.5972) (16.2541, 0.5895) (16.2765, 0.5821) (16.299, 0.5748) (16.3215, 0.5678) (16.344, 0.561) (16.3665, 0.5543) (16.389, 0.5479) (16.4115, 0.5417) (16.434, 0.5357) (16.4565, 0.53) (16.479, 0.5245) (16.5015, 0.5193) (16.524, 0.5143) (16.5464, 0.5095) (16.5689, 0.5049) (16.5914, 0.5006) (16.6138, 0.4965) (16.6362, 0.4927) (16.6587, 0.4891) (16.681, 0.486) (16.7034, 0.4832) (16.7258, 0.4808) (16.7481, 0.4787) (16.7704, 0.4769) (16.7926, 0.4753) (16.8149, 0.4738) (16.8371, 0.4726) (16.8592, 0.472) (16.8813, 0.4721) (16.8989, 0.473) (16.912, 0.4743) (16.9207, 0.4754) (16.9251, 0.4761) knots -1 -1 -1 -1 -1 -1 -0.98571429 -0.97142857 -0.95714286 -0.94285714 -0.92857143 -0.91428571 -0.9 -0.88571429 -0.87142857 -0.85714286 -0.84285714 -0.82857143 -0.81428571 -0.8 -0.78571429 -0.77142857 -0.75714286 -0.74285714 -0.72857143 -0.71428571 -0.7 -0.68571429 -0.67142857 -0.65714286 -0.64285714 -0.62857143 -0.61428571 -0.6 -0.58571429 -0.57142857 -0.55714286 -0.54285714 -0.52857143 -0.51428571 -0.5 -0.48571429 -0.47142857 -0.45714286 -0.44285714 -0.42857143 -0.41428571 -0.4 -0.38571429 -0.37142857 -0.35714286 -0.34285714 -0.32857143 -0.31428571 -0.3 -0.28571429 -0.27142857 -0.25714286 -0.24285714 -0.22857143 -0.21428571 -0.2 -0.18571429 -0.17142857 -0.15714286 -0.14285714 -0.12857143 -0.11428571 -0.1 -0.08571429 -0.07142857 -0.05714286 -0.04285714 -0.02857143 -0.01428571 0 0 0 0 0 0
  line L13 (16.9251, 0.4761) -> (17.7899, 0.6018)
  arc A27 (17.9029, 0.5192) -> (17.7899, 0.6018) centre (17.8043, 0.5028) ccw
  arc A28 (17.9029, 0.5192) -> (18.165, -0.4591) centre (23.0613, 1.3771) ccw
  arc A29 (18.1084, -0.5871) -> (18.165, -0.4591) centre (18.0714, -0.4942) ccw
  line L14 (18.1084, -0.5871) -> (17.2966, -0.9106)
  spline S14 degree 5 poles (17.2966, -0.9106) (17.2925, -0.9122) (17.2844, -0.9156) (17.2724, -0.9211) (17.2567, -0.9291) (17.2375, -0.94) (17.2187, -0.9517) (17.2001, -0.9638) (17.1815, -0.9761) (17.1631, -0.9887) (17.1447, -1.0014) (17.1264, -1.0144) (17.1082, -1.0276) (17.0902, -1.0412) (17.0724, -1.0551) (17.0548, -1.0694) (17.0373, -1.084) (17.0199, -1.0987) (17.0026, -1.1137) (16.9855, -1.1289) (16.9684, -1.1443) (16.9514, -1.1598) (16.9346, -1.1756) (16.9178, -1.1916) (16.9012, -1.2078) (16.8847, -1.2243) (16.8683, -1.2409) (16.8521, -1.2577) (16.8359, -1.2747) (16.8198, -1.2918) (16.8039, -1.3092) (16.788, -1.3267) (16.7723, -1.3444) (16.7566, -1.3623) (16.7411, -1.3803) (16.7257, -1.3985) (16.7103, -1.4169) (16.6951, -1.4354) (16.68, -1.4541) (16.665, -1.4729) (16.6501, -1.4919) (16.6353, -1.5111) (16.6206, -1.5304) (16.606, -1.5499) (16.5915, -1.5695) (16.5771, -1.5892) (16.5629, -1.6091) (16.5487, -1.6292) (16.5346, -1.6494) (16.5207, -1.6697) (16.5068, -1.6902) (16.493, -1.7108) (16.4794, -1.7315) (16.4659, -1.7524) (16.4524, -1.7734) (16.4391, -1.7946) (16.4259, -1.8159) (16.4127, -1.8373) (16.3997, -1.8588) (16.3868, -1.8805) (16.374, -1.9023) (16.3613, -1.9242) (16.3487, -1.9463) (16.3362, -1.9684) (16.3239, -1.9907) (16.3116, -2.0132) (16.2994, -2.0357) (16.2874, -2.0584) (16.2754, -2.0811) (16.2636, -2.104) (16.2518, -2.127) (16.2425, -2.1455) (16.2356, -2.1595) (16.231, -2.1688) (16.2287, -2.1734) knots 0 0 0 0 0 0 0.01428571 0.02857143 0.04285714 0.05714286 0.07142857 0.08571429 0.1 0.11428571 0.12857143 0.14285714 0.15714286 0.17142857 0.18571429 0.2 0.21428571 0.22857143 0.24285714 0.25714286 0.27142857 0.28571429 0.3 0.31428571 0.32857143 0.34285714 0.35714286 0.37142857 0.38571429 0.4 0.41428571 0.42857143 0.44285714 0.45714286 0.47142857 0.48571429 0.5 0.51428571 0.52857143 0.54285714 0.55714286 0.57142857 0.58571429 0.6 0.61428571 0.62857143 0.64285714 0.65714286 0.67142857 0.68571429 0.7 0.71428571 0.72857143 0.74285714 0.75714286 0.77142857 0.78571429 0.8 0.81428571 0.82857143 0.84285714 0.85714286 0.87142857 0.88571429 0.9 0.91428571 0.92857143 0.94285714 0.95714286 0.97142857 0.98571429 1 1 1 1 1 1
  arc A30 (16.2287, -2.1734) -> (16.5701, -2.7647) centre (23.0613, 1.3771) ccw
  spline S15 degree 5 poles (16.5701, -2.7647) (16.5753, -2.7651) (16.5856, -2.7658) (16.6012, -2.7667) (16.6219, -2.7679) (16.6476, -2.7693) (16.6734, -2.7705) (16.6991, -2.7715) (16.7247, -2.7724) (16.7503, -2.7731) (16.7759, -2.7737) (16.8014, -2.7741) (16.8268, -2.7744) (16.8522, -2.7745) (16.8776, -2.7745) (16.9029, -2.7743) (16.9281, -2.774) (16.9532, -2.7735) (16.9783, -2.7728) (17.0034, -2.772) (17.0284, -2.771) (17.0533, -2.7699) (17.0782, -2.7686) (17.1029, -2.7672) (17.1277, -2.7655) (17.1523, -2.7638) (17.1769, -2.7619) (17.2014, -2.7598) (17.2259, -2.7575) (17.2503, -2.7551) (17.2746, -2.7525) (17.2988, -2.7498) (17.3229, -2.7469) (17.347, -2.7438) (17.371, -2.7406) (17.3949, -2.7372) (17.4187, -2.7336) (17.4425, -2.7299) (17.4661, -2.7259) (17.4897, -2.7219) (17.5132, -2.7176) (17.5366, -2.7132) (17.5599, -2.7085) (17.583, -2.7038) (17.6061, -2.6988) (17.6291, -2.6936) (17.652, -2.6883) (17.6748, -2.6828) (17.6975, -2.6771) (17.7201, -2.6712) (17.7426, -2.6651) (17.7649, -2.6589) (17.7872, -2.6524) (17.8093, -2.6457) (17.8312, -2.6388) (17.8531, -2.6317) (17.8748, -2.6244) (17.8964, -2.6169) (17.9179, -2.6092) (17.9393, -2.6013) (17.9604, -2.5932) (17.9814, -2.5847) (18.0022, -2.576) (18.0227, -2.5669) (18.0431, -2.5575) (18.0633, -2.548) (18.0834, -2.5382) (18.1034, -2.5284) (18.1232, -2.5183) (18.1427, -2.5078) (18.1618, -2.4967) (18.1765, -2.4871) (18.1873, -2.4794) (18.1943, -2.474) (18.1977, -2.4713) knots -1 -1 -1 -1 -1 -1 -0.98571429 -0.97142857 -0.95714286 -0.94285714 -0.92857143 -0.91428571 -0.9 -0.88571429 -0.87142857 -0.85714286 -0.84285714 -0.82857143 -0.81428571 -0.8 -0.78571429 -0.77142857 -0.75714286 -0.74285714 -0.72857143 -0.71428571 -0.7 -0.68571429 -0.67142857 -0.65714286 -0.64285714 -0.62857143 -0.61428571 -0.6 -0.58571429 -0.57142857 -0.55714286 -0.54285714 -0.52857143 -0.51428571 -0.5 -0.48571429 -0.47142857 -0.45714286 -0.44285714 -0.42857143 -0.41428571 -0.4 -0.38571429 -0.37142857 -0.35714286 -0.34285714 -0.32857143 -0.31428571 -0.3 -0.28571429 -0.27142857 -0.25714286 -0.24285714 -0.22857143 -0.21428571 -0.2 -0.18571429 -0.17142857 -0.15714286 -0.14285714 -0.12857143 -0.11428571 -0.1 -0.08571429 -0.07142857 -0.05714286 -0.04285714 -0.02857143 -0.01428571 0 0 0 0 0 0
  line L15 (18.1977, -2.4713) -> (18.8838, -1.9301)
  arc A31 (19.023, -1.945) -> (18.8838, -1.9301) centre (18.9457, -2.0086) ccw
  arc A32 (19.023, -1.945) -> (19.7391, -2.6612) centre (23.0613, 1.3771) ccw
  arc A33 (19.7541, -2.8003) -> (19.7391, -2.6612) centre (19.6756, -2.7384) ccw
  line L16 (19.7541, -2.8003) -> (19.2128, -3.4864)
  spline S16 degree 5 poles (19.2128, -3.4864) (19.2101, -3.4899) (19.2047, -3.4969) (19.1971, -3.5076) (19.1875, -3.5224) (19.1763, -3.5414) (19.1659, -3.5609) (19.1558, -3.5808) (19.1459, -3.6007) (19.1362, -3.6208) (19.1266, -3.641) (19.1172, -3.6614) (19.1081, -3.682) (19.0994, -3.7027) (19.0909, -3.7237) (19.0828, -3.7449) (19.0749, -3.7662) (19.0672, -3.7877) (19.0597, -3.8093) (19.0525, -3.831) (19.0454, -3.8529) (19.0385, -3.8749) (19.0317, -3.897) (19.0253, -3.9192) (19.019, -3.9415) (19.0129, -3.964) (19.007, -3.9866) (19.0013, -4.0093) (18.9958, -4.0321) (18.9905, -4.055) (18.9853, -4.078) (18.9804, -4.1011) (18.9756, -4.1243) (18.971, -4.1476) (18.9665, -4.171) (18.9623, -4.1944) (18.9582, -4.218) (18.9543, -4.2417) (18.9505, -4.2654) (18.947, -4.2892) (18.9436, -4.3131) (18.9403, -4.3371) (18.9372, -4.3612) (18.9343, -4.3853) (18.9316, -4.4096) (18.929, -4.4339) (18.9266, -4.4582) (18.9244, -4.4827) (18.9223, -4.5072) (18.9203, -4.5318) (18.9186, -4.5565) (18.917, -4.5812) (18.9155, -4.606) (18.9142, -4.6308) (18.9131, -4.6558) (18.9121, -4.6807) (18.9113, -4.7058) (18.9107, -4.7309) (18.9102, -4.756) (18.9098, -4.7813) (18.9096, -4.8066) (18.9096, -4.8319) (18.9097, -4.8573) (18.91, -4.8827) (18.9104, -4.9082) (18.911, -4.9338) (18.9117, -4.9594) (18.9126, -4.985) (18.9137, -5.0107) (18.9149, -5.0365) (18.9162, -5.0623) (18.9174, -5.0829) (18.9184, -5.0985) (18.919, -5.1088) (18.9194, -5.114) knots 0 0 0 0 0 0 0.01428571 0.02857143 0.04285714 0.05714286 0.07142857 0.08571429 0.1 0.11428571 0.12857143 0.14285714 0.15714286 0.17142857 0.18571429 0.2 0.21428571 0.22857143 0.24285714 0.25714286 0.27142857 0.28571429 0.3 0.31428571 0.32857143 0.34285714 0.35714286 0.37142857 0.38571429 0.4 0.41428571 0.42857143 0.44285714 0.45714286 0.47142857 0.48571429 0.5 0.51428571 0.52857143 0.54285714 0.55714286 0.57142857 0.58571429 0.6 0.61428571 0.62857143 0.64285714 0.65714286 0.67142857 0.68571429 0.7 0.71428571 0.72857143 0.74285714 0.75714286 0.77142857 0.78571429 0.8 0.81428571 0.82857143 0.84285714 0.85714286 0.87142857 0.88571429 0.9 0.91428571 0.92857143 0.94285714 0.95714286 0.97142857 0.98571429 1 1 1 1 1 1
  arc A34 (18.9194, -5.114) -> (19.5107, -5.4554) centre (23.0613, 1.3771) ccw
  spline S17 degree 5 poles (19.5107, -5.4554) (19.5153, -5.4531) (19.5247, -5.4485) (19.5386, -5.4416) (19.5571, -5.4323) (19.5801, -5.4206) (19.603, -5.4087) (19.6258, -5.3968) (19.6484, -5.3847) (19.671, -5.3725) (19.6934, -5.3603) (19.7157, -5.3479) (19.7379, -5.3354) (19.7599, -5.3228) (19.7818, -5.3101) (19.8036, -5.2973) (19.8253, -5.2844) (19.8468, -5.2714) (19.8683, -5.2583) (19.8895, -5.245) (19.9107, -5.2317) (19.9317, -5.2183) (19.9526, -5.2047) (19.9733, -5.1911) (19.994, -5.1773) (20.0144, -5.1635) (20.0348, -5.1495) (20.0549, -5.1354) (20.075, -5.1213) (20.0949, -5.107) (20.1147, -5.0926) (20.1343, -5.0781) (20.1537, -5.0635) (20.173, -5.0488) (20.1922, -5.034) (20.2112, -5.0191) (20.23, -5.0041) (20.2487, -4.989) (20.2673, -4.9738) (20.2856, -4.9585) (20.3038, -4.943) (20.3219, -4.9275) (20.3397, -4.9119) (20.3574, -4.8961) (20.3749, -4.8803) (20.3923, -4.8643) (20.4094, -4.8482) (20.4264, -4.8321) (20.4432, -4.8158) (20.4599, -4.7994) (20.4763, -4.7829) (20.4925, -4.7663) (20.5085, -4.7496) (20.5243, -4.7327) (20.5399, -4.7157) (20.5552, -4.6987) (20.5704, -4.6815) (20.5854, -4.6642) (20.6002, -4.6468) (20.6147, -4.6293) (20.629, -4.6117) (20.6429, -4.5939) (20.6565, -4.5759) (20.6698, -4.5578) (20.6827, -4.5395) (20.6954, -4.5211) (20.708, -4.5026) (20.7203, -4.4841) (20.7325, -4.4654) (20.7441, -4.4466) (20.7551, -4.4274) (20.763, -4.4117) (20.7685, -4.3997) (20.7719, -4.3916) (20.7735, -4.3875) knots -1 -1 -1 -1 -1 -1 -0.98571429 -0.97142857 -0.95714286 -0.94285714 -0.92857143 -0.91428571 -0.9 -0.88571429 -0.87142857 -0.85714286 -0.84285714 -0.82857143 -0.81428571 -0.8 -0.78571429 -0.77142857 -0.75714286 -0.74285714 -0.72857143 -0.71428571 -0.7 -0.68571429 -0.67142857 -0.65714286 -0.64285714 -0.62857143 -0.61428571 -0.6 -0.58571429 -0.57142857 -0.55714286 -0.54285714 -0.52857143 -0.51428571 -0.5 -0.48571429 -0.47142857 -0.45714286 -0.44285714 -0.42857143 -0.41428571 -0.4 -0.38571429 -0.37142857 -0.35714286 -0.34285714 -0.32857143 -0.31428571 -0.3 -0.28571429 -0.27142857 -0.25714286 -0.24285714 -0.22857143 -0.21428571 -0.2 -0.18571429 -0.17142857 -0.15714286 -0.14285714 -0.12857143 -0.11428571 -0.1 -0.08571429 -0.07142857 -0.05714286 -0.04285714 -0.02857143 -0.01428571 0 0 0 0 0 0
  line L17 (20.7735, -4.3875) -> (21.0971, -3.5757)
  arc A35 (21.2251, -3.5191) -> (21.0971, -3.5757) centre (21.19, -3.6127) ccw
  arc A36 (21.2251, -3.5191) -> (22.2033, -3.7812) centre (23.0613, 1.3771) ccw
  arc A37 (22.2859, -3.8942) -> (22.2033, -3.7812) centre (22.1869, -3.8799) ccw
  line L18 (22.2859, -3.8942) -> (22.1602, -4.759)
  spline S18 degree 5 poles (22.1602, -4.759) (22.1595, -4.7634) (22.1584, -4.7721) (22.1571, -4.7853) (22.1562, -4.8028) (22.1561, -4.8249) (22.1568, -4.8471) (22.1579, -4.8693) (22.1594, -4.8915) (22.161, -4.9138) (22.1628, -4.9361) (22.1649, -4.9584) (22.1673, -4.9807) (22.1701, -5.0031) (22.1733, -5.0255) (22.1768, -5.0479) (22.1806, -5.0703) (22.1847, -5.0928) (22.1891, -5.1152) (22.1936, -5.1377) (22.1984, -5.1602) (22.2034, -5.1826) (22.2086, -5.2051) (22.2141, -5.2276) (22.2199, -5.2501) (22.2258, -5.2726) (22.232, -5.2951) (22.2385, -5.3176) (22.2451, -5.3401) (22.2519, -5.3626) (22.259, -5.3851) (22.2662, -5.4076) (22.2737, -5.4301) (22.2813, -5.4525) (22.2892, -5.475) (22.2972, -5.4975) (22.3055, -5.5199) (22.3139, -5.5424) (22.3225, -5.5648) (22.3313, -5.5872) (22.3403, -5.6096) (22.3495, -5.632) (22.3589, -5.6544) (22.3685, -5.6768) (22.3782, -5.6991) (22.3881, -5.7215) (22.3982, -5.7438) (22.4085, -5.7661) (22.419, -5.7883) (22.4296, -5.8106) (22.4404, -5.8328) (22.4514, -5.8551) (22.4625, -5.8773) (22.4738, -5.8994) (22.4853, -5.9216) (22.4969, -5.9437) (22.5088, -5.9658) (22.5207, -5.9879) (22.5329, -6.0099) (22.5452, -6.0319) (22.5577, -6.0539) (22.5703, -6.0759) (22.5831, -6.0978) (22.5961, -6.1197) (22.6092, -6.1416) (22.6225, -6.1634) (22.6359, -6.1852) (22.6495, -6.207) (22.6633, -6.2287) (22.6772, -6.2504) (22.6912, -6.2721) (22.7026, -6.2894) (22.7112, -6.3024) (22.717, -6.311) (22.7199, -6.3153) knots 0 0 0 0 0 0 0.01428571 0.02857143 0.04285714 0.05714286 0.07142857 0.08571429 0.1 0.11428571 0.12857143 0.14285714 0.15714286 0.17142857 0.18571429 0.2 0.21428571 0.22857143 0.24285714 0.25714286 0.27142857 0.28571429 0.3 0.31428571 0.32857143 0.34285714 0.35714286 0.37142857 0.38571429 0.4 0.41428571 0.42857143 0.44285714 0.45714286 0.47142857 0.48571429 0.5 0.51428571 0.52857143 0.54285714 0.55714286 0.57142857 0.58571429 0.6 0.61428571 0.62857143 0.64285714 0.65714286 0.67142857 0.68571429 0.7 0.71428571 0.72857143 0.74285714 0.75714286 0.77142857 0.78571429 0.8 0.81428571 0.82857143 0.84285714 0.85714286 0.87142857 0.88571429 0.9 0.91428571 0.92857143 0.94285714 0.95714286 0.97142857 0.98571429 1 1 1 1 1 1
  arc A38 (22.7199, -6.3153) -> (23.4026, -6.3153) centre (23.0613, 1.3771) ccw
  spline S19 degree 5 poles (23.4026, -6.3153) (23.4055, -6.311) (23.4113, -6.3024) (23.4199, -6.2894) (23.4313, -6.2721) (23.4453, -6.2504) (23.4592, -6.2287) (23.473, -6.207) (23.4866, -6.1852) (23.5, -6.1634) (23.5133, -6.1416) (23.5264, -6.1197) (23.5394, -6.0978) (23.5522, -6.0759) (23.5648, -6.0539) (23.5773, -6.0319) (23.5896, -6.0099) (23.6018, -5.9879) (23.6137, -5.9658) (23.6256, -5.9437) (23.6372, -5.9216) (23.6487, -5.8994) (23.66, -5.8773) (23.6711, -5.8551) (23.6821, -5.8328) (23.6929, -5.8106) (23.7035, -5.7883) (23.714, -5.7661) (23.7243, -5.7438) (23.7344, -5.7215) (23.7443, -5.6991) (23.754, -5.6768) (23.7636, -5.6544) (23.773, -5.632) (23.7822, -5.6096) (23.7912, -5.5872) (23.8, -5.5648) (23.8086, -5.5424) (23.817, -5.5199) (23.8253, -5.4975) (23.8333, -5.475) (23.8412, -5.4525) (23.8488, -5.4301) (23.8563, -5.4076) (23.8635, -5.3851) (23.8706, -5.3626) (23.8774, -5.3401) (23.884, -5.3176) (23.8905, -5.2951) (23.8967, -5.2726) (23.9026, -5.2501) (23.9084, -5.2276) (23.9139, -5.2051) (23.9191, -5.1826) (23.9241, -5.1602) (23.9289, -5.1377) (23.9334, -5.1152) (23.9378, -5.0928) (23.9419, -5.0703) (23.9457, -5.0479) (23.9492, -5.0255) (23.9524, -5.0031) (23.9552, -4.9807) (23.9576, -4.9584) (23.9597, -4.9361) (23.9615, -4.9138) (23.9631, -4.8915) (23.9646, -4.8693) (23.9657, -4.8471) (23.9664, -4.8249) (23.9663, -4.8028) (23.9654, -4.7853) (23.9641, -4.7721) (23.963, -4.7634) (23.9623, -4.759) knots -1 -1 -1 -1 -1 -1 -0.98571429 -0.97142857 -0.95714286 -0.94285714 -0.92857143 -0.91428571 -0.9 -0.88571429 -0.87142857 -0.85714286 -0.84285714 -0.82857143 -0.81428571 -0.8 -0.78571429 -0.77142857 -0.75714286 -0.74285714 -0.72857143 -0.71428571 -0.7 -0.68571429 -0.67142857 -0.65714286 -0.64285714 -0.62857143 -0.61428571 -0.6 -0.58571429 -0.57142857 -0.55714286 -0.54285714 -0.52857143 -0.51428571 -0.5 -0.48571429 -0.47142857 -0.45714286 -0.44285714 -0.42857143 -0.41428571 -0.4 -0.38571429 -0.37142857 -0.35714286 -0.34285714 -0.32857143 -0.31428571 -0.3 -0.28571429 -0.27142857 -0.25714286 -0.24285714 -0.22857143 -0.21428571 -0.2 -0.18571429 -0.17142857 -0.15714286 -0.14285714 -0.12857143 -0.11428571 -0.1 -0.08571429 -0.07142857 -0.05714286 -0.04285714 -0.02857143 -0.01428571 0 0 0 0 0 0
  line L19 (23.9623, -4.759) -> (23.8366, -3.8942)
  arc A39 (23.9192, -3.7812) -> (23.8366, -3.8942) centre (23.9356, -3.8799) ccw
  arc A40 (23.9192, -3.7812) -> (24.8974, -3.5191) centre (23.0613, 1.3771) ccw
  arc A41 (25.0254, -3.5757) -> (24.8974, -3.5191) centre (24.9326, -3.6127) ccw
  line L20 (25.0254, -3.5757) -> (25.349, -4.3875)
  spline S20 degree 5 poles (25.349, -4.3875) (25.3506, -4.3916) (25.354, -4.3997) (25.3595, -4.4117) (25.3674, -4.4274) (25.3784, -4.4466) (25.39, -4.4654) (25.4022, -4.4841) (25.4145, -4.5026) (25.4271, -4.5211) (25.4398, -4.5395) (25.4527, -4.5578) (25.466, -4.5759) (25.4796, -4.5939) (25.4935, -4.6117) (25.5078, -4.6293) (25.5223, -4.6468) (25.5371, -4.6642) (25.5521, -4.6815) (25.5673, -4.6987) (25.5826, -4.7157) (25.5982, -4.7327) (25.614, -4.7496) (25.63, -4.7663) (25.6462, -4.7829) (25.6626, -4.7994) (25.6793, -4.8158) (25.6961, -4.8321) (25.7131, -4.8482) (25.7302, -4.8643) (25.7476, -4.8803) (25.7651, -4.8961) (25.7828, -4.9119) (25.8006, -4.9275) (25.8187, -4.943) (25.8369, -4.9585) (25.8552, -4.9738) (25.8738, -4.989) (25.8925, -5.0041) (25.9113, -5.0191) (25.9303, -5.034) (25.9495, -5.0488) (25.9688, -5.0635) (25.9882, -5.0781) (26.0078, -5.0926) (26.0276, -5.107) (26.0475, -5.1213) (26.0676, -5.1354) (26.0877, -5.1495) (26.1081, -5.1635) (26.1286, -5.1773) (26.1492, -5.1911) (26.1699, -5.2047) (26.1908, -5.2183) (26.2118, -5.2317) (26.233, -5.245) (26.2542, -5.2583) (26.2757, -5.2714) (26.2972, -5.2844) (26.3189, -5.2973) (26.3407, -5.3101) (26.3626, -5.3228) (26.3846, -5.3354) (26.4068, -5.3479) (26.4291, -5.3603) (26.4515, -5.3725) (26.4741, -5.3847) (26.4967, -5.3968) (26.5195, -5.4087) (26.5424, -5.4206) (26.5654, -5.4323) (26.5839, -5.4416) (26.5978, -5.4485) (26.6072, -5.4531) (26.6118, -5.4554) knots 0 0 0 0 0 0 0.01428571 0.02857143 0.04285714 0.05714286 0.07142857 0.08571429 0.1 0.11428571 0.12857143 0.14285714 0.15714286 0.17142857 0.18571429 0.2 0.21428571 0.22857143 0.24285714 0.25714286 0.27142857 0.28571429 0.3 0.31428571 0.32857143 0.34285714 0.35714286 0.37142857 0.38571429 0.4 0.41428571 0.42857143 0.44285714 0.45714286 0.47142857 0.48571429 0.5 0.51428571 0.52857143 0.54285714 0.55714286 0.57142857 0.58571429 0.6 0.61428571 0.62857143 0.64285714 0.65714286 0.67142857 0.68571429 0.7 0.71428571 0.72857143 0.74285714 0.75714286 0.77142857 0.78571429 0.8 0.81428571 0.82857143 0.84285714 0.85714286 0.87142857 0.88571429 0.9 0.91428571 0.92857143 0.94285714 0.95714286 0.97142857 0.98571429 1 1 1 1 1 1
  arc A42 (26.6118, -5.4554) -> (27.2031, -5.114) centre (23.0613, 1.3771) ccw